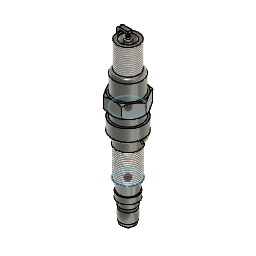
gyakorlati 11 gyujtogyertya (Autodesk Fusion 360 design; units mm, degrees)
Autodesk Fusion 360 part; units mm, degrees
sketch "Sketch1" plane through (0, 0, 0) normal (0, 0, 1) x (1, 0, 0)
  line L0 (-23.094, 40) -> (-46.188, 0)
  line L1 (-46.188, 0) -> (-23.094, -40)
  line L2 (-23.094, -40) -> (23.094, -40)
  line L3 (23.094, -40) -> (46.188, 0)
  line L4 (46.188, 0) -> (23.094, 40)
  line L5 (23.094, 40) -> (-23.094, 40)
  circle A0 centre (0, 0) radius 32.3702
  circle A1 centre (0, 0) radius 25
  constraint coincident A0.centre A1.centre
extrude "Extrude1" add sketch "Sketch1" along normal blind 35 contours L0 L1 L2 L3 L4 L5 | A0 makes body 1
thread "Thread1" "ISO Metric profile 50.0 M50x4 6H" major diameter 50.4462 minor diameter 45.9699 pitch 4 angle 60 resizes the face on face at (24.8758, -2.4892, 23.3333) on bodies 1
sketch "Sketch2" plane through (0, 0, 0) normal (0, 1, 0) x (1, 0, 0)
  line L0 (-40, 0) -> (-50, 0)
  line L1 (-50, 0) -> (-50, -10)
  line L2 (-50, -10) -> (-40, 0)
  constraint horizontal L0
  constraint perpendicular L0 L1
revolve "Revolve1" cut sketch "Sketch2" angle 360 about axis through (0, 0, 1.75) along (0, 0, 1) bodies 1
sketch "Sketch3" plane through (0, 0, 0) normal (0, 1, 0) x (1, 0, 0)
  line L0 (-40, -35) -> (-49, -35)
  line L1 (-49, -29) -> (-40, -35)
  line L2 (-49, -35) -> (-49, -29)
  constraint horizontal L0
  constraint perpendicular L0 L2
revolve "Revolve2" cut sketch "Sketch3" angle 360 about axis through (0, 0, 1.75) along (0, 0, 1) bodies 1
fillet "Fillet1" radius 0.5 1 edges at (-21.4295, 8.3117, 35) on bodies 1
fillet "Fillet2" radius 0.5 1 edges at (-21.4295, 8.3117, 0) on bodies 1
sketch "Sketch4" plane through (0, 0, 0) normal (0, 0, 1) x (1, 0, 0)
  circle A0 centre (0, 0) radius 23
  constraint coincident A0.centre origin
extrude "Extrude2" add sketch "Sketch4" along normal blind 150 bodies 1
ref_plane "WorkPlane1" through (0, 0, 150) normal (0, 0, 1) x (1, 0, 0)
sketch "Sketch5" plane through (0, 0, 150) normal (0, 0, 1) x (1, 0, 0)
  circle A0 centre (0, 0) radius 23.0217
  constraint coincident A0.centre origin
extrude "Extrude3" add sketch "Sketch5" along normal blind 175 bodies 1
thread "Thread2" "ISO Metric profile 45.0 M45x4.5 6g" major diameter 44.687 minor diameter 39.5358 pitch 4.5 angle 60 resizes the face on face at (22.9931, -1.1475, 266.6667) on bodies 1
delete_face "DeleteFace1" 1 faces at (-22.2325, -2.2247, 208.3333) on bodies 1
extrude "Extrude4" cut 1 faces at (10.6672, -7.6452, 0) along direction (0, 0, 1) blind 150 on bodies 1 bodies 1
sketch "Sketch6" plane through (0, 0, 0) normal (0, 0, 1) x (1, 0, 0)
  circle A0 centre (0, 0) radius 35
  constraint coincident A0.centre origin
extrude "Extrude5" cut sketch "Sketch6" along normal blind 35 bodies 1
extrude "Extrude6" add sketch "Sketch6" along normal blind 70 bodies 1
sketch "Sketch7" plane through (0, 0, 70) normal (0, 0, 1) x (-1, 0, 0)
  circle A0 centre (0, 0) radius 35
  circle A1 centre (0, 0) radius 35
  constraint concentric A0 A1
extrude "Extrude7" add sketch "Sketch7" 1 faces at (8.8451, -11.8425, 70) along normal blind 15 on bodies 1 bodies 1
fillet "Fillet3" radius 10 1 faces at (-2.7189, -2.1683, 85) on bodies 1
sketch "Sketch8" plane through (0, 0, 85) normal (0, 0, 1) x (-1, 0, 0)
  circle A0 centre (0, 0) radius 25
  circle A1 centre (0, 0) radius 25
  constraint concentric A0 A1
sketch "Sketch9" plane through (0, 0, 85) normal (0, 0, 1) x (-1, 0, 0)
  circle A0 centre (0, 0) radius 22.6984
  constraint coincident A0.centre origin
extrude "Extrude8" add sketch "Sketch8" along normal blind 5 bodies 1
extrude "Extrude9" cut sketch "Sketch9" along normal blind 5 bodies 1
extrude "Extrude10" add 1 faces at (-6.0992, 2.2302, 85) along direction (0, 0, 1) blind 65 on bodies 1 bodies 1
extrude "Extrude11" add 1 faces at (-24.0552, 2.3697, 90) along direction (0, 0, 1) blind 60 on bodies 1 bodies 1
thread "Thread3" "ISO Metric profile 55.0 M55x4 6g" major diameter 54.7025 minor diameter 50.1258 pitch 4 angle 60 resizes the face on face at (-24.9689, 1.2461, 128.3333) on bodies 1
sketch "Sketch10" plane through (0, 0, 150) normal (0, 0, 1) x (-1, 0, 0)
  circle A0 centre (0, 0) radius 27.3513
  circle A1 centre (0, 0) radius 19
  constraint concentric A0 A1
extrude "Extrude12" cut sketch "Sketch10" against normal blind 8 contours A1 bodies 1
sketch "Sketch11" plane through (0, 0, 142) normal (0, 0, 1) x (-1, 0, 0)
  circle A0 centre (0, 0) radius 19
  circle A1 centre (0, 0) radius 9
  constraint coincident A0.centre A1.centre
extrude "Extrude13" add sketch "Sketch11" along normal blind 9 draft -9 contours A1 bodies 1
fillet "Fillet4" radius 4 1 edges at (7.062, -2.7391, 151) on bodies 1
extrude "Extrude14" add 1 faces at (-0.2623, -1.9665, 151) along direction (0, 0, 1) blind 6 on bodies 1 bodies 1
sketch "Sketch12" plane through (0, 0, 150) normal (0, 0, 1) x (-1, 0, 0)
  circle A0 centre (0, 0) radius 19
  circle A1 centre (0, 0) radius 27.3513
  line L0 (24.8975, 4.1666) -> (20.4669, 4.1666)
  line L1 (20.4669, 4.1666) -> (20.4669, -6.327)
  line L2 (20.4669, -6.327) -> (24.8975, -6.327)
  line L3 (24.8975, -6.327) -> (24.8975, 4.1666)
  constraint horizontal L0
  constraint vertical L1
  constraint horizontal L2
  constraint vertical L3
extrude "Extrude15" add sketch "Sketch12" along normal blind 15 contours L0 L1 L2 L3 bodies 1
sketch "Sketch13" plane through (-20.4669, 0, 0) normal (1, 0, 0) x (0, 1, 0)
  line L0 (-4.1666, 150) -> (6.327, 150)
  line L1 (6.327, 150) -> (6.327, 165)
  line L2 (6.327, 165) -> (-4.1666, 165)
  line L3 (-4.1666, 165) -> (-4.1666, 150)
  line L4 (-4.1666, 165) -> (6.327, 165)
  line L5 (6.327, 165) -> (6.327, 160.2652)
  line L6 (6.327, 160.2652) -> (-4.1666, 160.2652)
  line L7 (-4.1666, 160.2652) -> (-4.1666, 165)
  constraint horizontal L4
  constraint vertical L5
  constraint horizontal L6
  constraint vertical L7
  constraint coincident L1 L5.end
  constraint coincident L2.end L3.start
extrude "Extrude16" add sketch "Sketch13" along normal blind 20 contours L1 L2 L3 L4 L5 L6 L7 bodies 1
fillet "Fillet5" radius 7.5 2 edges at (-20.4669, 1.0802, 160.2652) (-24.8975, 1.0802, 165) on bodies 1
extrude "Extrude17" cut 1 faces at (-15.5959, 0.9439, 142) along direction (0, 0, -1) blind 60 on bodies 1 bodies 1
fillet "Fillet6" radius 1 1 edges at (3.8768, 1.5037, 157) on bodies 1
delete_face "DeleteFace2" 1 faces at (-11.754, 2.8291, 165) on bodies 1
delete_face "DeleteFace3" 1 faces at (-23.3952, -4.1666, 153.7775) on bodies 1
sketch "Sketch14" plane through (0, 0, 150) normal (0, 0, 1) x (-1, 0, 0)
  circle A0 centre (0, 0) radius 19
  circle A1 centre (0, 0) radius 27.3513
  line L0 (25, 5) -> (20, 5)
  line L1 (20, 5) -> (20, -5)
  line L2 (20, -5) -> (25, -5)
  line L3 (25, -5) -> (25, 5)
  constraint horizontal L0
  constraint vertical L1
  constraint horizontal L2
  constraint vertical L3
extrude "Extrude18" add sketch "Sketch14" along normal blind 20 contours L0 L1 L2 L3 bodies 1
sketch "Sketch15" plane through (-20, 0, 0) normal (1, 0, 0) x (0, 1, 0)
  line L0 (-5, 150) -> (5, 150)
  line L1 (5, 150) -> (5, 170)
  line L2 (5, 170) -> (-5, 170)
  line L3 (-5, 170) -> (-5, 150)
  line L4 (-5, 170) -> (5, 170)
  line L5 (5, 170) -> (5, 163.5215)
  line L6 (5, 163.5215) -> (-5, 163.5215)
  line L7 (-5, 163.5215) -> (-5, 170)
  constraint horizontal L4
  constraint vertical L5
  constraint horizontal L6
  constraint vertical L7
  constraint coincident L1 L5.end
  constraint coincident L2.end L3.start
extrude "Extrude19" add sketch "Sketch15" along normal blind 25 contours L1 L2 L3 L4 L5 L6 L7 bodies 1
fillet "Fillet7" radius 7.5 2 edges at (-20, 0, 163.5215) (-25, 0, 170) on bodies 1
extrude "Extrude20" add sketch "Sketch6" against normal blind 20 bodies 1
sketch "Sketch16" plane through (0, 0, -20) normal (0, 0, -1) x (1, 0, 0)
  circle A0 centre (0, 0) radius 35
  circle A1 centre (0, 0) radius 40
  constraint coincident A0.centre A1.centre
extrude "Extrude21" add sketch "Sketch16" along normal blind 20 separate body makes body 2
extrude "Extrude22" add sketch "Sketch6" against normal blind 40 bodies 1 2
extrude "Extrude23" add 1 faces at (9.4847, 14.2223, -40) along direction (0, 0, -1) blind 10 on bodies 1 bodies 1
coil "CoilPrimitive1" add diameter 70 section circle size 8 on centre turns 1 pitch 10 right hand placed x (1, 0, 0) y (0, -1, 0) z (0, 0, -1) at (0, 0, -50) bodies 1
sketch "Sketch18" plane through (0, 0, -50) normal (0, 0, -1) x (1, 0, 0)
  spline S0 degree 3 poles (31, 0) (31, 4.121) (30.1951, 8.2013) (27.0651, 15.8355) (24.7681, 19.3125) (18.9568, 25.2205) (15.4936, 27.5854) (7.8151, 30.897) (3.6726, 31.7939) (-4.804, 31.9967) (-9.0359, 31.278) (-18.0251, 27.9954) (-21.6813, 25.401) (-25.6393, 22.2951) (-26.7879, 21.2811) (-27.7555, 20.6661) (-27.951, 20.5682) (-28.1427, 20.5336) (-28.1874, 20.5303) (-28.2563, 20.5421) (-28.282, 20.5509) (-28.3259, 20.5785) (-28.3432, 20.595) (-28.3749, 20.6386) (-28.3872, 20.666) (-28.4109, 20.744) (-28.4157, 20.7996) (-28.4158, 20.9824) (-28.3854, 21.1327) (-28.2545, 21.6332) (-28.0449, 22.1373) (-26.7654, 24.557) (-24.6962, 27.4276) (-18.0015, 32.9451) (-13.9689, 35.1757) (-4.7791, 37.9713) (0.0597, 38.4358) (9.731, 37.4866) (14.4739, 36.0447) (23.185, 31.4058) (27.0631, 28.2344) (33.0355, 21.0111) (35.2361, 17.1491) (38.2325, 8.8298) (39, 4.4312) (39, 0) knots 0 0 0 0 1.236307 1.236307 2.475128 2.475128 3.72186 3.72186 4.982338 4.982338 6.262266 6.262266 7.84207 7.84207 8.849917 8.849917 9.156832 9.156832 9.242277 9.242277 9.297415 9.297415 9.346382 9.346382 9.4058 9.4058 9.51034 9.51034 9.773871 9.773871 10.553494 10.553494 12.98193 12.98193 15.337341 15.337341 17.695378 17.695378 20.100196 20.100196 22.530219 22.530219 24.690604 24.690604 26.860631 26.860631 26.860631 26.860631
  line L0 (39, 0) -> (31, 0)
  circle A0 centre (0, 0) radius 40
  circle A1 centre (0, 0) radius 30
  constraint concentric A0 A1
extrude "Extrude24" add sketch "Sketch18" along normal blind 30 contours A1 bodies 1
sketch "Sketch19" plane through (0, 0, -80) normal (0, 0, -1) x (1, 0, 0)
  circle A0 centre (0, 0) radius 30
  circle A1 centre (0, 0) radius 28.5304
  constraint concentric A0 A1
extrude "Extrude25" add sketch "Sketch19" along normal blind 80 contours A1 bodies 1
thread "Thread4" "ISO Metric profile 58.0 M58x4 6g" major diameter 57.7025 minor diameter 53.1258 pitch 4 angle 60 resizes the face on face at (28.4949, 1.4221, -133.3333) on bodies 1
extrude "Extrude26" cut 1 faces at (-2.8587, 5.8836, -160) along direction (0, 0, 1) blind 5 on bodies 1 bodies 1
sketch "Sketch20" plane through (0, 0, -155) normal (0, 0, -1) x (1, 0, 0)
  circle A0 centre (0, 0) radius 28.8513
  circle A1 centre (0, 0) radius 28.8513
  constraint coincident A0.centre A1.centre
sketch "Sketch21" plane through (0, 0, -155) normal (0, 0, -1) x (1, 0, 0)
  circle A0 centre (0, 0) radius 27.1214
  constraint coincident A0.centre origin
extrude "Extrude27" add sketch "Sketch21" along normal blind 28 draft -10 bodies 1
sketch "Sketch22" plane through (0, 0, -183) normal (0, 0, -1) x (1, 0, 0)
  circle A0 centre (0, 0) radius 22.1842
  circle A1 centre (0, 0) radius 25
  constraint coincident A0.centre A1.centre
extrude "Extrude28" add sketch "Sketch22" along normal blind 15 separate body makes body 3
sketch "Sketch23" plane through (0, 0, -183) normal (0, 0, -1) x (1, 0, 0)
  circle A0 centre (0, 0) radius 22.1842
  circle A1 centre (0, 0) radius 20
  constraint concentric A0 A1
extrude "Extrude29" add sketch "Sketch23" along normal blind 30 contours A1 bodies 1
sketch "Sketch24" plane through (0, 0, -213) normal (0, 0, -1) x (1, 0, 0)
  circle A0 centre (0, 0) radius 20
  circle A1 centre (0, 0) radius 17.3955
  constraint concentric A0 A1
extrude "Extrude30" add sketch "Sketch24" along normal blind 20 draft 15 contours A1 bodies 1
extrude "Extrude31" add 1 faces at (1.5378, -1.6574, -233) along direction (0, 0, -1) blind 20 draft -15 on bodies 1 bodies 1
fillet "Fillet8" radius 50 1 edges at (-21.2146, -8.2284, -233) on bodies 1
extrude "Extrude32" add 1 faces at (2.1184, -5.3977, -253) along direction (0, 0, -1) blind 10 draft -50 on bodies 1 bodies 1
